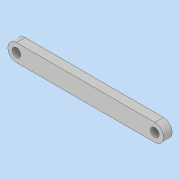
# Autodesk Inventor part: Part3
Saved by Autodesk Inventor 2017 (Build 210142000, 142)
## iProperties
Created: 2016-10-24
Part Number: Part3
Material: Generic
Document SubType Name: Modeling
Designer: techn
Density: 1 g/cm^3
Appearance: Default
Author: techn
Autodesk Inventor part; units mm, degrees
ref_plane "YZ Plane" through (0, 0, 0) normal (1, 0, 0) x (0, 1, 0)
ref_plane "XZ Plane" through (0, 0, 0) normal (0, 1, 0) x (-1, 0, 0)
ref_plane "XY Plane" through (0, 0, 0) normal (0, 0, 1) x (1, 0, 0)
sketch "Sketch1" plane through (0, 0, 0) normal (0, 0, 1) x (1, 0, 0)
  line L0 (0, 0) -> (-50.8, 0)
  line L1 (-50.8, 0) -> (-50.8, 6.35)
  line L2 (-50.8, 6.35) -> (0, 6.35)
  line L3 (0, 6.35) -> (0, 0)
  arc A0 (-50.8, 6.35) -> (-50.8, 0) centre (-50.8, 3.175) ccw
  arc A1 (0, 0) -> (0, 6.35) centre (0, 3.175) ccw
  circle A2 centre (-50.8, 3.175) radius 1.5875
  circle A3 centre (0, 3.175) radius 1.5875
  dimension "d0" = 50.8
  dimension "d1" = 6.35
  dimension "d2" = 3.175
  dimension "d3" = 3.175
  dimension "d4" = 3.175
  constraints: 8 end point, 4 centre point, 4 point on circle, 2 coincident, 2 parallel, 2 tangent, 1 horizontal, 1 perpendicular
  measures "d0" distance of L1.end L2.end
  measures "d1" distance of L0.end L1.end
  measures "d2" radius of A1
  measures "d3" diameter of A2
  measures "d4" diameter of A3
extrude "Extrusion1" add sketch "Sketch1" along normal blind 3.175
extrude "Extrusion2" cut sketch "Sketch1" along normal blind 3.175 contours A3 L3 | L3 A3 | A2 L1 | L1 A2
body "Solid1"
